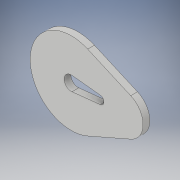
# Autodesk Inventor part: Pata - Soporte Antebrazo
Saved by Autodesk Inventor 2019 (Build 230136000, 136)
## iProperties
Created: 2020-02-11
Part Number: Pata - Soporte Antebrazo
Material: Generic
Document SubType Name: Modeling
Designer: jacqu
Density: 1 g/cm^3
Appearance: Default
radio_muslo: 20.000 mm
Author: jacqu
Autodesk Inventor part; units mm, degrees
ref_plane "YZ Plane" through (0, 0, 0) normal (1, 0, 0) x (0, 1, 0)
ref_plane "XZ Plane" through (0, 0, 0) normal (0, 1, 0) x (-1, 0, 0)
ref_plane "XY Plane" through (0, 0, 0) normal (0, 0, 1) x (1, 0, 0)
sketch "Sketch1" plane through (0, 0, 0) normal (0, 0, 1) x (1, 0, 0)
  line L0 (0.3684, -3.4604) -> (14.1917, -1.9888)
  arc A0 (0.3684, 3.4604) -> (0.3684, -3.4604) centre (0, 0) ccw
  line L1 (0.3684, 3.4604) -> (14.1917, 1.9888)
  arc A1 (14.1917, -1.9888) -> (14.1917, 1.9888) centre (13.98, 0) ccw
  line L2 (8, -18.3303) -> (29, -9.1652)
  line L3 (8, 18.3303) -> (29, 9.1652)
  arc A2 (29, -9.1652) -> (29, 9.1652) centre (25, 0) ccw
  arc A3 (8, 18.3303) -> (8, -18.3303) centre (0, 0) ccw
  dimension "d13" = 3.48
  dimension "d14" = 2
  dimension "d15" = 19.46
  dimension "d17" = 20
  dimension "d18" = 10
  dimension "d19" = 25
  constraints: 8 end point, 8 point on circle, 7 tangent, 4 centre point, 3 coincident, 2 horizontal alignment, 1 equal length
  measures "d13" radius of A0
  measures "d14" radius of A1
  measures "d17" radius of A3
  measures "d18" radius of A2
  measures "d19" distance of point (0, 0) A2.centre
extrude "Extrusion2" add sketch "Sketch1" along normal blind 3.3
equation "\"d17\" = radio_muslo"
equation "\"d18\" = 0.5 * radio_muslo"
equation "\"radio_muslo\" = 20"
body "Solid2"
